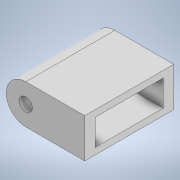
# Autodesk Inventor part: 1st arm
Saved by Autodesk Inventor 2022 (Build 260153000, 153)
## iProperties
Created: 2021-06-29
Part Number: 1st arm
Material: Generic
Document SubType Name: Modeling
Designer: USER
Density: 1 g/cm^3
Appearance: Default
Author: USER
Autodesk Inventor part; units mm, degrees
ref_plane "YZ Plane" through (0, 0, 0) normal (1, 0, 0) x (0, 1, 0)
ref_plane "XZ Plane" through (0, 0, 0) normal (0, 1, 0) x (-1, 0, 0)
ref_plane "XY Plane" through (0, 0, 0) normal (0, 0, 1) x (1, 0, 0)
sketch "Sketch1" plane through (0, 0, 0) normal (0, 0, 1) x (1, 0, 0)
  line L0 (0, 0) -> (60, 0)
  line L1 (60, 0) -> (60, -30)
  line L2 (60, -30) -> (0, -30)
  line L3 (0, -30) -> (0, 0)
  dimension "d0" = 60
  dimension "d1" = 30
  constraints: 8 end point, 2 parallel, 1 horizontal, 1 perpendicular
  measures "d0" distance of L1.end L2.end
  measures "d1" distance of L0.end L1.end
extrude "Extrusion1" add sketch "Sketch1" along normal blind 68
sketch "Sketch2" plane through (0, 0, 68) normal (0, 0, 1) x (1, 0, 0)
  circle A0 centre (15, -15) radius 5
  line L0 (0, -30) -> (60, -30) projected
  line L1 (0, 0) -> (0, -30) projected
  dimension "d4" = 10
  dimension "d5" = 15
  dimension "d6" = 15
  constraints: 1 centre point
  measures "d4" diameter of A0
  measures "d5" distance from line of L0 A0.centre
  measures "d6" distance from line of L1 A0.centre
extrude "Extrusion2" cut sketch "Sketch2" against normal blind 68
sketch "Sketch3" plane through (60, -30, 0) normal (1, 0, 0) x (0, 0, -1)
  line L0 (-60, 5) -> (-8, 5)
  line L1 (-8, 5) -> (-8, 25)
  line L2 (-8, 25) -> (-60, 25)
  line L3 (-60, 25) -> (-60, 5)
  line L4 (-60, 5) -> (-8, 25) construction
  line L5 (-8, 5) -> (-60, 25) construction
  line L6 (-68, 0) -> (-68, 30) projected
  line L7 (0, 0) -> (-68, 0) projected
  point P0 (0, 30)
  point P1 (-34, 15)
  dimension "d9" = 52
  dimension "d10" = 20
  dimension "d11" = 34
  dimension "d12" = 15
  constraints: 12 end point, 2 midpoint, 2 parallel, 1 horizontal, 1 perpendicular
  measures "d9" distance of L2.end L1.end
  measures "d10" distance of L1.end L0.end
  measures "d11" distance from line of L6 point (-34, 15)
  measures "d12" distance from line of L7 point (-34, 15)
extrude "Extrusion3" cut sketch "Sketch3" against normal blind 52
full round fillet "Full Round Fillet1" first side at (42.6667, -5, 25.3333) centre faces at (8, -11.6667, 42.6667) second side at (42.6667, -25, 42.6667)
fillet "Fillet1" radius 15 2 edges at (0, 0, 34) (0, -30, 34)
body "Solid1"
